Autodesk Inventor part; units mm, degrees
(part 2 of 2)
sketch "Sketch7" plane through (50.9518, -3.7878, 59.6125) normal (0, 0, -1) x (-1, 0, 0)
  circle A0 centre (50.9518, 123.3878) radius 9.525 projected
  line L0 (128.7396, 142.7878) -> (122.0761, 142.7878) projected
  line L1 (122.0761, 142.7878) -> (122.0761, 148.7878) projected
  line L2 (-20.1725, 148.7878) -> (122.0761, 148.7878) projected
  line L3 (-20.1725, 148.7878) -> (-20.1725, 142.7878) projected
  line L4 (-20.1725, 142.7878) -> (-26.8359, 142.7878) projected
  line L5 (-26.8359, 142.7878) -> (-26.8359, 70.8342) projected
  arc A1 (-26.8359, 56.7413) -> (-26.8359, 70.8342) centre (-23.0482, 63.7878) ccw projected
  line L6 (-26.8359, 56.7413) -> (-26.8359, 50.8342) projected
  arc A2 (-26.8359, 36.7413) -> (-26.8359, 50.8342) centre (-23.0482, 43.7878) ccw projected
  line L7 (-26.8359, 36.7413) -> (-26.8359, 28.6734) projected
  line L8 (-26.8359, 28.6734) -> (-25.5366, 25.5366) projected
  line L9 (-25.5366, 25.5366) -> (0, 0) projected
  line L10 (0, 0) -> (33.9053, 0) projected
  arc A3 (47.9983, 0) -> (33.9053, 0) centre (40.9518, 3.7878) ccw projected
  line L11 (47.9983, 0) -> (53.9053, 0) projected
  arc A4 (67.9983, 0) -> (53.9053, 0) centre (60.9518, 3.7878) ccw projected
  line L12 (67.9983, 0) -> (100.0661, 0) projected
  line L13 (100.0661, 0) -> (103.2029, 1.2993) projected
  line L14 (103.2029, 1.2993) -> (128.7396, 26.8359) projected
  line L15 (128.7396, 26.8359) -> (128.7396, 36.7413) projected
  arc A5 (128.7396, 50.8342) -> (128.7396, 36.7413) centre (124.9518, 43.7878) ccw projected
  line L16 (128.7396, 50.8342) -> (128.7396, 56.7413) projected
  arc A6 (128.7396, 70.8342) -> (128.7396, 56.7413) centre (124.9518, 63.7878) ccw projected
  line L17 (128.7396, 142.7878) -> (128.7396, 70.8342) projected
  circle A7 centre (-23.0482, 63.7878) radius 2.63 construction
  line L18 (50.9518, 123.3878) -> (-23.0482, 63.7878) construction
  circle A8 centre (124.9518, 63.7878) radius 2.63 construction
  line L19 (-23.0482, 63.7878) -> (124.9518, 63.7878) construction
  line L20 (124.9518, 63.7878) -> (50.9518, 123.3878) construction
  line L21 (50.9518, 123.3878) -> (50.9518, 43.7878) construction
  line L22 (50.9518, 43.7878) -> (40.9518, 3.7878) construction
  circle A9 centre (60.9518, 3.7878) radius 2.63 construction
  line L23 (50.9518, 43.7878) -> (60.9518, 3.7878) construction
  circle A10 centre (124.9518, 43.7878) radius 2.63 construction
  line L24 (60.9518, 3.7878) -> (124.9518, 43.7878) construction
  circle A11 centre (-23.0482, 43.7878) radius 2.63 construction
  line L25 (-23.0482, 43.7878) -> (40.9518, 3.7878) construction
  line L26 (-23.0482, 43.7878) -> (124.9518, 43.7878) construction
  line L27 (52.7185, -2.7122) -> (69.1851, -2.7122) construction
  line L28 (50.9518, 123.3878) -> (-20.1725, 148.7878) construction
  line L29 (50.9518, 123.3878) -> (122.0761, 148.7878) construction
  circle A12 centre (50.9518, 123.3878) radius 12.7 construction
  line L30 (6.5311, 142.6227) -> (38.3175, 131.2711)
  line L31 (63.5861, 131.2711) -> (95.3725, 142.6227)
  arc A13 (7.5989, 148.7878) -> (6.5311, 142.6227) centre (7.5989, 145.6128) ccw
  arc A14 (95.3725, 142.6227) -> (94.3047, 148.7878) centre (94.3047, 145.6128) ccw
  arc A15 (60.205, 132.0865) -> (41.6986, 132.0865) centre (50.9518, 123.3878) ccw
  arc A16 (38.3175, 131.2711) -> (41.6986, 132.0865) centre (39.3853, 134.2612) ccw
  arc A17 (60.205, 132.0865) -> (63.5861, 131.2711) centre (62.5183, 134.2612) ccw
  line L32 (122.0761, 145.4164) -> (65.7217, 125.291)
  line L33 (36.1819, 125.291) -> (-20.1725, 145.4164)
  line L34 (64.2748, 116.7341) -> (121.2246, 70.8664)
  line L35 (44.6018, 60.6128) -> (-15.7052, 60.6128)
  line L36 (-19.3209, 70.8664) -> (37.6288, 116.7341)
  arc A18 (63.2034, 120.043) -> (63.622, 122.5183) centre (50.9518, 123.3878) ccw
  arc A19 (65.7217, 125.291) -> (63.622, 122.5183) centre (66.7896, 122.301) ccw
  arc A20 (63.2034, 120.043) -> (64.2748, 116.7341) centre (66.2663, 119.2068) ccw
  arc A21 (38.2816, 122.5183) -> (38.7002, 120.043) centre (50.9518, 123.3878) ccw
  arc A22 (38.2816, 122.5183) -> (36.1819, 125.291) centre (35.114, 122.301) ccw
  arc A23 (37.6288, 116.7341) -> (38.7002, 120.043) centre (35.6373, 119.2068) ccw
  line L37 (60.2917, 111.7886) -> (108.9357, 72.6105)
  line L38 (44.6018, 66.9628) -> (-5.0406, 66.9628)
  line L39 (-7.0321, 72.6105) -> (41.6119, 111.7886)
  line L40 (47.7768, 70.1378) -> (47.7768, 108.8381)
  arc A24 (-7.0321, 72.6105) -> (-5.0406, 66.9628) centre (-5.0406, 70.1378) ccw
  arc A25 (44.6018, 66.9628) -> (47.7768, 70.1378) centre (44.6018, 70.1378) ccw
  arc A26 (45.0731, 112.1303) -> (45.8718, 111.748) centre (50.9518, 123.3878) ccw
  arc A27 (45.0731, 112.1303) -> (41.6119, 111.7886) centre (43.6034, 109.3159) ccw
  arc A28 (47.7768, 108.8381) -> (45.8718, 111.748) centre (44.6018, 108.8381) ccw
  line L41 (54.1268, 70.1378) -> (54.1268, 108.8381)
  arc A29 (56.0318, 111.748) -> (56.8305, 112.1303) centre (50.9518, 123.3878) ccw
  arc A30 (60.2917, 111.7886) -> (56.8305, 112.1303) centre (58.3002, 109.3159) ccw
  arc A31 (56.0318, 111.748) -> (54.1268, 108.8381) centre (57.3018, 108.8381) ccw
  line L42 (106.9442, 66.9628) -> (57.3018, 66.9628)
  arc A32 (54.1268, 70.1378) -> (57.3018, 66.9628) centre (57.3018, 70.1378) ccw
  arc A33 (106.9442, 66.9628) -> (108.9357, 72.6105) centre (106.9442, 70.1378) ccw
  line L43 (47.7768, 50.1378) -> (47.7768, 57.4378)
  arc A34 (47.7768, 57.4378) -> (44.6018, 60.6128) centre (44.6018, 57.4378) ccw
  line L44 (-15.7052, 46.9628) -> (44.6018, 46.9628)
  arc A35 (44.6018, 46.9628) -> (47.7768, 50.1378) centre (44.6018, 50.1378) ccw
  line L45 (117.6088, 60.6128) -> (57.3018, 60.6128)
  line L46 (54.1268, 50.1378) -> (54.1268, 57.4378)
  arc A36 (57.3018, 60.6128) -> (54.1268, 57.4378) centre (57.3018, 57.4378) ccw
  line L47 (57.3018, 46.9628) -> (117.6088, 46.9628)
  arc A37 (54.1268, 50.1378) -> (57.3018, 46.9628) centre (57.3018, 50.1378) ccw
  line L48 (45.8991, 36.6677) -> (40.1018, 13.4788)
  line L49 (34.8367, 11.3538) -> (-2.5898, 34.7454)
  line L50 (-0.907, 40.6128) -> (42.8189, 40.6128)
  arc A38 (-0.907, 40.6128) -> (-2.5898, 34.7454) centre (-0.907, 37.4378) ccw
  arc A39 (45.8991, 36.6677) -> (42.8189, 40.6128) centre (42.8189, 37.4378) ccw
  arc A40 (34.8367, 11.3538) -> (37.7788, 11.1316) centre (36.5195, 14.0462) ccw
  arc A41 (38.1383, 11.2767) -> (40.1018, 13.4788) centre (37.0216, 14.2488) ccw
  line L51 (-18.5041, 37.2036) -> (31.4712, 5.969)
  arc A42 (32.9602, 3.4218) -> (31.4712, 5.969) centre (29.7885, 3.2766) ccw
  arc A43 (29.7936, 0) -> (32.9638, 3.3491) centre (29.7936, 3.175) ccw
  line L52 (56.0045, 36.6677) -> (61.8018, 13.4788)
  line L53 (67.0669, 11.3538) -> (104.4934, 34.7454)
  line L54 (102.8106, 40.6128) -> (59.0847, 40.6128)
  arc A44 (59.0847, 40.6128) -> (56.0045, 36.6677) centre (59.0847, 37.4378) ccw
  arc A45 (64.1248, 11.1316) -> (67.0669, 11.3538) centre (65.3841, 14.0462) ccw
  arc A46 (61.8018, 13.4788) -> (63.7653, 11.2767) centre (64.882, 14.2488) ccw
  line L55 (120.4077, 37.2036) -> (70.4324, 5.969)
  arc A47 (70.4324, 5.969) -> (68.9434, 3.4218) centre (72.1151, 3.2766) ccw
  arc A48 (68.9398, 3.3491) -> (72.11, 0) centre (72.11, 3.175) ccw
  arc A49 (104.4934, 34.7454) -> (102.8106, 40.6128) centre (102.8106, 37.4378) ccw
  line L56 (56.0907, 10.1414) -> (50.9518, 30.6969)
  line L57 (50.9518, 30.6969) -> (45.8129, 10.1414)
  point P0 (50.9518, 3.7878)
  point P1 (40.4392, 130.5134)
  point P2 (61.4644, 130.5134)
  point P3 (38.3036, 124.5333)
  point P4 (39.3834, 118.1473)
  point P5 (62.5202, 118.1473)
  point P6 (63.6, 124.5333)
  point P7 (117.6088, 60.6128)
  point P8 (58.5371, 113.2018)
  point P9 (115.948, 66.9628)
  point P10 (43.3665, 113.2018)
  point P11 (47.7768, 111.091)
  point P12 (54.1268, 111.091)
  point P13 (63.7653, 11.2767)
  point P14 (64.1248, 11.1316)
  dimension "d26" = 3.175
  dimension "d27" = 3.175
  dimension "d28" = 3.175
  dimension "d29" = 3.175
  dimension "d30" = 3.175
  dimension "d31" = 3.175
  dimension "d32" = 3.175
  dimension "d33" = 3.175
  dimension "d34" = 3.175
  dimension "d35" = 3.175
  dimension "d36" = 3.175
  dimension "d37" = 3.175
  dimension "d38" = 3.175
  dimension "d39" = 3.175
  dimension "d40" = 3.175
  dimension "d41" = 3.175
  dimension "d42" = 3.175
  dimension "d43" = 3.175
  dimension "d44" = 3.175
  dimension "d45" = 3.175
  dimension "d46" = 3.175
  dimension "d47" = 3.175
  dimension "d48" = 3.175
  dimension "d49" = 3.175
  dimension "d50" = 3.175
  dimension "d51" = 3.175
  dimension "d52" = 3.175
  dimension "d53" = 3.175
  constraints: 98 point on circle, 78 end point, 54 tangent, 37 centre point, 20 point on line, 18 symmetric about line, 10 equal radius, 4 collinear, 2 horizontal, 1 midpoint, 1 parallel, 1 vertical, 31 other
  measures "d27" distance between parallel lines of L28 L30
  measures "d28" radius of A13
  measures "d29" radius of A16
  measures "d30" distance between parallel lines of L32 L29
  measures "d31" distance between parallel lines of L20 L34
  measures "d32" radius of A19
  measures "d33" radius of A20
  measures "d34" radius of A22
  measures "d35" radius of A23
  measures "d36" distance between parallel lines of L37 L20
  measures "d37" distance between parallel lines of L21 L40
  measures "d38" radius of A24
  measures "d39" radius of A27
  measures "d40" distance between parallel lines of L21 L41
  measures "d41" radius of A30
  measures "d42" distance between parallel lines of L19 L42
  measures "d43" radius of A32
  measures "d44" radius of A34
  measures "d45" distance between parallel lines of L26 L44
  measures "d46" radius of A35
  measures "d47" radius of A36
  measures "d48" radius of A37
  measures "d49" distance between parallel lines of L50 L26
  measures "d50" radius of A38
  measures "d51" radius of A39
  measures "d52" distance between parallel lines of L51 L25
  measures "d53" distance between parallel lines of L56 L23
extrude "Extrusion6" add sketch "Sketch7" along normal blind 6.35 contours L32 A19 A18 A20 L34 A6 L45 A36 L46 A37 L47 A5 L55 A47 A4 A45 L53 A49 L54 A44 L52 A46 L56 L57 A3 A41 L48 A39 L50 A38 L49 A40 A42 L51 A2 L44 A35 L43 A34 L35 A1 L36 A23 A21 A22 L33 L3 L2 A13 L30 A16 A15 A17 L31 A14 L1
fillet "Fillet2" radius 1.5875 17 edges at (43.3529, 145, 56.4375) (-43.3529, 145, 56.4375) (-71.1243, 145, 56.4375) (-71.1243, 141.6286, 56.4375) (71.1243, 145, 56.4375) (71.1243, 141.6286, 56.4375) (70.2728, 67.0787, 56.4375) (-70.2728, 67.0787, 56.4375) (-66.657, 56.825, 56.4375) (-66.657, 43.175, 56.4375) (66.657, 56.825, 56.4375) (66.657, 43.175, 56.4375) (69.4559, 33.4158, 56.4375) (0, 26.9091, 56.4375) (5.1389, 6.3537, 56.4375) (-5.1389, 6.3537, 56.4375) (-69.4559, 33.4158, 56.4375)
equation "\"d21\" = 0.5 * d20"
equation "\"d30\" = d27"
equation "\"d31\" = d30"
equation "\"d36\" = d31"
equation "\"d37\" = d31"
equation "\"d40\" = d37"
equation "\"d42\" = d36"
equation "\"d45\" = d42"
equation "\"d49\" = d45"
body "Solid1"
